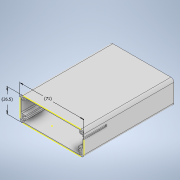
# Autodesk Inventor part: case
Saved by Autodesk Inventor 2021 (Build 250183000, 183)
## iProperties
Created: 2025-06-24
Part Number: case
Material: Generic
Document SubType Name: Modeling
Designer: Toby
Density: 1 g/cm^3
Appearance: Default
Author: Toby
Autodesk Inventor part; units mm, degrees
ref_plane "YZ Plane" through (0, 0, 0) normal (1, 0, 0) x (0, 1, 0)
ref_plane "XZ Plane" through (0, 0, 0) normal (0, 1, 0) x (-1, 0, 0)
ref_plane "XY Plane" through (0, 0, 0) normal (0, 0, 1) x (1, 0, 0)
sketch "Sketch1" plane through (0, 0, 0) normal (0, 0, 1) x (1, 0, 0)
  line L0 (-35.5, 13.25) -> (35.5, 13.25)
  line L1 (35.5, 13.25) -> (35.5, -13.25)
  line L2 (35.5, -13.25) -> (-35.5, -13.25)
  line L3 (-35.5, -13.25) -> (-35.5, 13.25)
  line L4 (-34.3, 12.05) -> (34.3, 12.05)
  line L5 (34.3, 12.05) -> (34.3, -12.05)
  line L6 (34.3, -12.05) -> (-34.3, -12.05)
  line L7 (-34.3, -12.05) -> (-34.3, 12.05)
  point P0 (0, 0)
  dimension "d0" = 71
  dimension "d1" = 26.5
  dimension "d2" = 35.5
  dimension "d3" = 13.25
  dimension "d4" = 1.2
  dimension "d5" = 1.2
  dimension "d6" = 1.2
  dimension "d7" = 1.2
  constraints: 16 end point, 4 parallel, 2 horizontal, 2 perpendicular
  measures "d0" distance of L0.start L0.end
  measures "d1" distance of L2.end L0.start
  measures "d2" distance from line of point (0, 0) L3
  measures "d3" distance from line of point (0, 0) L0
  measures "d4" distance between parallel lines of L4 L0
  measures "d5" distance between parallel lines of L2 L6
  measures "d6" distance between parallel lines of L7 L3
  measures "d7" distance between parallel lines of L1 L5
extrude "Extrusion1" add sketch "Sketch1" along normal blind 100
fillet "Fillet1" radius 2 4 edges at (-34.3, 12.05, 50) (34.3, 12.05, 50) (34.3, -12.05, 50) (-34.3, -12.05, 50)
fillet "Fillet2" radius 3.25 4 edges at (-35.5, 13.25, 50) (-35.5, -13.25, 50) (35.5, -13.25, 50) (35.5, 13.25, 50)
sketch "Sketch2" plane through (0, 0, 100) normal (0, 0, 1) x (1, 0, 0)
  line L0 (-34.3, -10.05) -> (-34.3, 10.05) projected
  line L1 (-34.3, -7.9) -> (-31.3, -7.9)
  line L2 (-31.3, -7.9) -> (-31.3, -9.4)
  line L3 (-31.3, -9.4) -> (-34.3, -9.4)
  line L4 (-34.3, -9.4) -> (-34.3, -7.9)
  line L5 (34.3, 10.05) -> (34.3, -10.05) projected
  line L6 (34.3, -7.9) -> (31.3, -7.9)
  line L7 (31.3, -7.9) -> (31.3, -9.4)
  line L8 (31.3, -9.4) -> (34.3, -9.4)
  line L9 (34.3, -9.4) -> (34.3, -7.9)
  line L10 (-32.25, -13.25) -> (32.25, -13.25) projected
  line L11 (-34.3, -6.05) -> (-31.3, -6.05)
  line L12 (-31.3, -6.05) -> (-31.3, -4.55)
  line L13 (-31.3, -4.55) -> (-34.3, -4.55)
  line L14 (-34.3, -4.55) -> (-34.3, -6.05)
  line L15 (31.3, -6.05) -> (34.3, -6.05)
  line L16 (34.3, -6.05) -> (34.3, -4.55)
  line L17 (34.3, -4.55) -> (31.3, -4.55)
  line L18 (31.3, -4.55) -> (31.3, -6.05)
  point P0 (0, 0)
  dimension "d12" = 3.85
  dimension "d13" = 1.5
  dimension "d14" = 3
  dimension "d15" = 3
  dimension "d16" = 1.5
  dimension "d17" = 1.85
  constraints: 32 end point, 8 parallel, 5 collinear, 5 point on line, 4 horizontal, 4 perpendicular
  measures "d12" distance between parallel lines of L10 L3
  measures "d13" distance between parallel lines of L3 L1
  measures "d14" distance between parallel lines of L0 L2
  measures "d15" distance of L6.start L6.end
  measures "d16" distance between parallel lines of L11 L13
  measures "d17" distance between parallel lines of L1 L11
extrude "Extrusion2" add sketch "Sketch2" against normal blind 100
fillet "Fillet3" radius 1 4 edges at (-34.3, -4.55, 50) (-34.3, -9.4, 50) (34.3, -9.4, 50) (34.3, -4.55, 50)
sketch "Sketch3" plane through (0, 0, 100) normal (0, 0, 1) x (1, 0, 0)
  line L0 (32.25, 13.25) -> (-32.25, 13.25) projected
  line L1 (-35.5, 10) -> (-35.5, -10) projected
  line L2 (-32.25, -13.25) -> (32.25, -13.25) projected
  line L3 (35.5, -10) -> (35.5, 10) projected
  circle A0 centre (-32.5, 10.25) radius 2
  circle A1 centre (-32.5, -10.25) radius 2
  circle A2 centre (32.5, -10.25) radius 2
  circle A3 centre (32.5, 10.25) radius 2
  point P0 (0, 0)
  dimension "d21" = 3
  dimension "d22" = 3
  dimension "d23" = 3
  dimension "d24" = 3
  dimension "d25" = 3
  dimension "d26" = 3
  dimension "d27" = 3
  dimension "d28" = 3
  dimension "d29" = 4
  dimension "d30" = 4
  dimension "d31" = 4
  dimension "d32" = 4
  constraints: 4 centre point, 4 coincident
  measures "d21" distance from line of L0 point (-32.5, 10.25)
  measures "d22" distance from line of L1 point (-32.5, 10.25)
  measures "d23" distance from line of L1 point (-32.5, -10.25)
  measures "d24" distance from line of L2 point (-32.5, -10.25)
  measures "d25" distance from line of L2 point (32.5, -10.25)
  measures "d26" distance from line of L3 point (32.5, -10.25)
  measures "d27" distance from line of L0 point (32.5, 10.25)
  measures "d28" distance from line of L3 point (32.5, 10.25)
  measures "d29" diameter of A0
  measures "d30" diameter of A1
  measures "d31" diameter of A2
  measures "d32" diameter of A3
extrude "Extrusion3" add sketch "Sketch3" against normal blind 100
sketch "Sketch4" plane through (0, 0, 100) normal (0, 0, 1) x (1, 0, 0)
  arc A0 (-34.3, 9.3782) -> (-31.6282, 12.05) centre (-32.5, 10.25) ccw projected
  arc A1 (31.6282, 12.05) -> (34.3, 9.3782) centre (32.5, 10.25) ccw projected
  arc A2 (31.3, -8.65) -> (31.6282, -12.05) centre (32.5, -10.25) ccw projected
  arc A3 (-31.6282, -12.05) -> (-31.3, -8.65) centre (-32.5, -10.25) ccw projected
  circle A4 centre (-32.5, 10.25) radius 1
  circle A5 centre (-32.5, -10.25) radius 1
  circle A6 centre (32.5, 10.25) radius 1
  circle A7 centre (32.5, -10.25) radius 1
  point P0 (0, 0)
  dimension "d35" = 2
  dimension "d36" = 2
  dimension "d37" = 2
  dimension "d38" = 2
  constraints: 8 coincident, 4 centre point
  measures "d35" diameter of A4
  measures "d36" diameter of A5
  measures "d37" diameter of A6
  measures "d38" diameter of A7
extrude "Extrusion4" cut sketch "Sketch4" against normal blind 100
sketch "Sketch5" plane through (35.5, -10, 0) normal (1, 0, 0) x (0, 0, -1)
  line L0 (-100, 20) -> (-100, 0) projected
  line L1 (-100, 17) -> (-75, 17)
  line L2 (-75, 17) -> (-75, 14.9)
  line L3 (-75, 14.9) -> (-100, 14.9)
  line L4 (-100, 14.9) -> (-100, 17)
  line L5 (-100, 20) -> (0, 20) projected
  point P0 (0, 10)
  dimension "d41" = 2.1
  dimension "d42" = 3
  dimension "d43" = 25
  constraints: 8 end point, 2 parallel, 1 horizontal, 1 perpendicular, 1 point on line
  measures "d41" distance between parallel lines of L3 L1
  measures "d42" distance between parallel lines of L5 L1
  measures "d43" distance between parallel lines of L0 L2
extrude "Extrusion5" cut sketch "Sketch5" against normal blind 2
sketch "Sketch6" plane through (0, 0, 100) normal (0, 0, 1) x (1, 0, 0)
  line L0 (34.3, -6.05) -> (34.3, -7.9) projected
  line L1 (-34.3, -7.9) -> (-34.3, -6.05) projected
  line L2 (-31.3, -7.9) -> (-34.3, -7.9) projected
  line L3 (-31.3, -7.9) -> (-29.5, -7.9)
  line L4 (-29.5, -7.9) -> (-29.5, -9.4)
  line L5 (-29.5, -9.4) -> (-31.3, -9.4)
  line L6 (-31.3, -9.4) -> (-31.3, -7.9)
  line L7 (-31.3, -6.05) -> (-31.3, -4.55) projected
  line L8 (-31.3, -4.55) -> (-29.5, -4.55)
  line L9 (-29.5, -4.55) -> (-29.5, -6.05)
  line L10 (-29.5, -6.05) -> (-31.3, -6.05)
  line L11 (-31.3, -6.05) -> (-31.3, -4.55)
  line L12 (31.3, -4.55) -> (29.5, -4.55)
  line L13 (29.5, -4.55) -> (29.5, -6.05)
  line L14 (29.5, -6.05) -> (31.3, -6.05)
  line L15 (31.3, -6.05) -> (31.3, -4.55)
  line L16 (31.3, -7.9) -> (29.5, -7.9)
  line L17 (29.5, -7.9) -> (29.5, -9.4)
  line L18 (29.5, -9.4) -> (31.3, -9.4)
  line L19 (31.3, -9.4) -> (31.3, -7.9)
  line L20 (-31.3, -6.05) -> (-34.3, -6.05) projected
  line L21 (-34.3, -6.05) -> (-32.5, -6.05)
  line L22 (-32.5, -6.05) -> (-32.5, -7.9)
  line L23 (-32.5, -7.9) -> (-34.3, -7.9)
  line L24 (-34.3, -7.9) -> (-34.3, -6.05)
  line L25 (34.3, -6.05) -> (31.3, -6.05) projected
  line L26 (31.3, -7.9) -> (34.3, -7.9) projected
  line L27 (34.3, -6.05) -> (32.5, -6.05)
  line L28 (32.5, -6.05) -> (32.5, -7.9)
  line L29 (32.5, -7.9) -> (34.3, -7.9)
  line L30 (34.3, -7.9) -> (34.3, -6.05)
  point P0 (0, 0)
  dimension "d46" = 68.6
  dimension "d47" = 65
  dimension "d48" = 1.8
  dimension "d49" = 1.8
  dimension "d50" = 3
  dimension "d51" = 1.5
  dimension "d52" = 3
  constraints: 48 end point, 12 parallel, 8 point on line, 6 horizontal, 6 perpendicular
  measures "d46" distance between parallel lines of L0 L1
  measures "d47" distance between parallel lines of L28 L22
  measures "d48" distance between parallel lines of L0 L28
  measures "d49" distance between parallel lines of L1 L22
  measures "d50" distance between parallel lines of L9 L22
  measures "d51" distance between parallel lines of L3 L5
  measures "d52" distance between parallel lines of L28 L13
extrude "Extrusion6" add sketch "Sketch6" against normal blind 100
sketch "Sketch7" plane through (0, 0, 100) normal (0, 0, 1) x (1, 0, 0)
  line L0 (-32.25, -13.25) -> (32.25, -13.25) projected
  line L1 (32.25, 13.25) -> (-32.25, 13.25) projected
  line L2 (35.5, -10) -> (35.5, 4.9) projected
  line L3 (-35.5, 10) -> (-35.5, -10) projected
  point P0 (0, 0)
  dimension "d55" = 26.5
  dimension "d56" = 71
  measures "d55" distance between parallel lines of L0 L1
  measures "d56" distance between parallel lines of L2 L3
body "Solid1"
